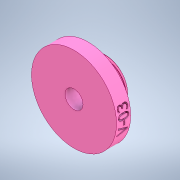
# Autodesk Inventor part: brakeHandle
Saved by Autodesk Inventor 2021.1 (Build 251245010, 245A)
## iProperties
Created: 2020-08-18
Part Number: brakeHandle
Material: Polycarbonate, Smoke
Document SubType Name: Modeling
Designer: robst
Density: 1.2 g/cm^3
Appearance: Pink
innerDiameter: 0.635 in
heightOfBrake: 0.250 in
majorDiameter: 1.623 in
pitchDiameter: 1.569 in
minorDiameter: 1.524 in
pitch: 0.083 in
crestFlat: 0.017 in
rootRadius: 0.009 in
threadsPerInch: 12.000 ul
threadDepth: 0.060 in
Author: robst
Autodesk Inventor part; units mm, degrees
ref_plane "XZ Plane" through (0, 0, 0) normal (0, 1, 0) x (-1, 0, 0)
ref_plane "XY Plane" through (0, 0, 0) normal (0, 0, 1) x (1, 0, 0)
sketch "Sketch1" plane through (0, 0, 0) normal (0, 0, 1) x (1, 0, 0)
  circle A0 centre (0, 0) radius 8.0645
  circle A1 centre (0, 0) radius 20.5061
  dimension "d0" = 16.129
  dimension "d1" = 41.0121
  constraints: 2 centre point, 2 coincident
  measures "d0" diameter of A0
  measures "d1" diameter of A1
extrude "Extrusion1" add sketch "Sketch1" against normal blind 15.24
sketch "Sketch2" plane through (0, 0, 0) normal (0, 0, 1) x (1, 0, 0)
  circle A0 centre (0, 0) radius 8.0645
  circle A1 centre (0, 0) radius 38.1
  dimension "d4" = 76.2
  dimension "d56" = 16.129
  constraints: 2 centre point, 2 coincident
  measures "d4" diameter of A1
  measures "d56" diameter of A0
extrude "Extrusion2" add sketch "Sketch2" along normal blind 12.7
sketch "Sketch9" plane through (0, 0, 0) normal (1, 0, 0) x (0, 1, 0)
  line L0 (20.5061, 0) -> (20.5061, -15.24) projected
  line L1 (-20.5061, -15.24) -> (20.5061, -15.24) projected
  line L2 (20.5061, -17.3567) -> (19.3002, -18.0529)
  line L3 (19.3002, -18.44) -> (20.5061, -19.1362)
  arc A0 (19.3002, -18.0529) -> (19.3002, -18.44) centre (19.412, -18.2464) ccw
  line L4 (20.5061, -17.3567) -> (20.5061, -19.1362)
  line L5 (0, -15.24) -> (0, -43.7839) construction
  point P0 (0, 0)
  dimension "d38" = 60
  dimension "d39" = 0.2235
  dimension "d41" = 2.1167
  dimension "d42" = 20.506
  dimension "d52" = 19.1884
  constraints: 8 end point, 2 point on circle, 2 tangent, 2 vertical, 1 centre point, 1 equal length, 1 midpoint
  measures "d38" angle of L3 L2
  measures "d39" radius of A0
  measures "d41" distance from line of L2.start L1
  measures "d42" distance from line of L4 point (0, 0)
  measures "d52" distance edge to line of A0 L5
coil "Coil2" sketch "Sketch9" operation cut axis through (0, 0, -10) along (0, 0, 1) pitch 2.1167 turns 9.2 hand right
ref_plane "Work Plane1" through (38.1, 0, 0) normal (1, 0, 0) x (0, 1, 0)
sketch "Sketch10" plane through (38.1, 0, 0) normal (1, 0, 0) x (0, 1, 0)
  line L0 (38.1, 0) -> (38.1, 12.7) construction
  line L1 (38.1, 6.35) -> (-38.1, 6.35) construction
  line L2 (-38.1, 0) -> (-38.1, 12.7) construction
  line L3 (-5.1906, 10.795) -> (-8.2524, 1.905)
  line L4 (-8.2524, 1.905) -> (-9.5276, 1.905)
  line L5 (-9.5276, 1.905) -> (-12.5894, 10.795)
  line L6 (-12.5894, 10.795) -> (-11.3214, 10.795)
  line L7 (-11.3214, 10.795) -> (-8.8576, 3.4107)
  line L8 (-8.8576, 3.4107) -> (-6.3937, 10.795)
  line L9 (-6.3937, 10.795) -> (-5.1906, 10.795)
  line L10 (-1.2355, 5.255) -> (-4.5999, 5.255)
  line L11 (-4.5999, 5.255) -> (-4.5999, 6.3356)
  line L12 (-4.5999, 6.3356) -> (-1.2355, 6.3356)
  line L13 (-1.2355, 6.3356) -> (-1.2355, 5.255)
  spline S0 degree 2 poles (5.4788, 6.35) (5.4788, 3.9582) (4.0884, 1.7177) (2.6403, 1.7177) knots 0 0 0 1 2 2 2
  spline S1 degree 2 poles (2.6403, 1.7177) (1.1707, 1.7177) (-0.2053, 4.0014) (-0.2053, 6.3428) knots 0 0 0 1 2 2 2
  spline S2 degree 2 poles (-0.2053, 6.3428) (-0.2053, 8.749) (1.1851, 10.9751) (2.6403, 10.9751) knots 0 0 0 1 2 2 2
  spline S3 degree 2 poles (2.6403, 10.9751) (4.1028, 10.9751) (5.4788, 8.6698) (5.4788, 6.35) knots 0 0 0 1 2 2 2
  spline S4 degree 2 poles (3.9515, 3.6412) (4.1244, 4.0807) (4.2685, 5.4351) (4.2685, 6.35) knots 0 0 0 1 2 2 2
  spline S5 degree 2 poles (4.2685, 6.35) (4.2685, 7.2649) (4.1244, 8.6121) (3.9443, 9.066) knots 0 0 0 1 2 2 2
  spline S6 degree 2 poles (3.9443, 9.066) (3.7642, 9.5199) (3.1374, 9.9881) (2.6403, 9.9881) knots 0 0 0 1 2 2 2
  spline S7 degree 2 poles (2.6403, 9.9881) (2.1433, 9.9881) (1.5021, 9.5199) (1.3148, 9.0516) knots 0 0 0 1 2 2 2
  spline S8 degree 2 poles (1.3148, 9.0516) (1.1347, 8.5977) (1.005, 7.2145) (1.005, 6.3428) knots 0 0 0 1 2 2 2
  spline S9 degree 2 poles (1.005, 6.3428) (1.005, 5.4062) (1.1203, 4.1527) (1.3076, 3.6628) knots 0 0 0 1 2 2 2
  spline S10 degree 2 poles (1.3076, 3.6628) (1.4805, 3.2018) (2.1216, 2.7047) (2.6403, 2.7047) knots 0 0 0 1 2 2 2
  spline S11 degree 2 poles (2.6403, 2.7047) (3.1302, 2.7047) (3.7714, 3.1729) (3.9515, 3.6412) knots 0 0 0 1 2 2 2
  spline S12 degree 2 poles (9.0161, 9.9521) (8.6919, 9.9521) (8.0507, 9.7936) (7.7409, 9.6711) knots 0 0 0 1 2 2 2
  spline S13 degree 2 poles (7.7409, 9.6711) (7.4528, 9.5487) (7.0277, 9.2893) (6.862, 9.1741) knots 0 0 0 1 2 2 2
  line L14 (6.862, 9.1741) -> (6.79, 9.1741)
  line L15 (6.79, 9.1741) -> (6.79, 10.4348)
  spline S14 degree 2 poles (6.79, 10.4348) (7.179, 10.6437) (8.5118, 10.9823) (9.1097, 10.9823) knots 0 0 0 1 2 2 2
  spline S15 degree 2 poles (9.1097, 10.9823) (9.7149, 10.9823) (10.6154, 10.7374) (10.9828, 10.478) knots 0 0 0 1 2 2 2
  spline S16 degree 2 poles (10.9828, 10.478) (11.3719, 10.1971) (11.7753, 9.383) (11.7753, 8.8355) knots 0 0 0 1 2 2 2
  spline S17 degree 2 poles (11.7753, 8.8355) (11.7753, 8.1006) (10.8099, 6.9912) (10.1327, 6.8471) knots 0 0 0 1 2 2 2
  line L16 (10.1327, 6.8471) -> (10.1327, 6.7606)
  spline S18 degree 2 poles (10.1327, 6.7606) (10.4137, 6.703) (11.0549, 6.4437) (11.3286, 6.1843) knots 0 0 0 1 2 2 2
  spline S19 degree 2 poles (11.3286, 6.1843) (11.6024, 5.9322) (11.9482, 5.1253) (11.9482, 4.5417) knots 0 0 0 1 2 2 2
  spline S20 degree 2 poles (11.9482, 4.5417) (11.9482, 3.9438) (11.5375, 2.928) (11.1629, 2.539) knots 0 0 0 1 2 2 2
  spline S21 degree 2 poles (11.1629, 2.539) (10.7739, 2.1355) (9.6717, 1.7177) (8.9728, 1.7177) knots 0 0 0 1 2 2 2
  spline S22 degree 2 poles (8.9728, 1.7177) (8.3029, 1.7177) (6.9917, 2.0419) (6.545, 2.2652) knots 0 0 0 1 2 2 2
  line L17 (6.545, 2.2652) -> (6.545, 3.5259)
  line L18 (6.545, 3.5259) -> (6.6315, 3.5259)
  spline S23 degree 2 poles (6.6315, 3.5259) (7.0061, 3.2522) (8.274, 2.7479) (8.9008, 2.7479) knots 0 0 0 1 2 2 2
  spline S24 degree 2 poles (8.9008, 2.7479) (9.2682, 2.7479) (10.0031, 2.9784) (10.248, 3.245) knots 0 0 0 1 2 2 2
  spline S25 degree 2 poles (10.248, 3.245) (10.4857, 3.5115) (10.7379, 4.1455) (10.7379, 4.6282) knots 0 0 0 1 2 2 2
  spline S26 degree 2 poles (10.7379, 4.6282) (10.7379, 5.1109) (10.4569, 5.7376) (10.2048, 5.9177) knots 0 0 0 1 2 2 2
  spline S27 degree 2 poles (10.2048, 5.9177) (9.9526, 6.0979) (9.2682, 6.2347) (8.8648, 6.2347) knots 0 0 0 1 2 2 2
  line L19 (8.8648, 6.2347) -> (8.3605, 6.2347)
  line L20 (8.3605, 6.2347) -> (8.3605, 7.2217)
  line L21 (8.3605, 7.2217) -> (8.7567, 7.2217)
  spline S28 degree 2 poles (8.7567, 7.2217) (9.5564, 7.2217) (10.565, 7.9854) (10.565, 8.713) knots 0 0 0 1 2 2 2
  spline S29 degree 2 poles (10.565, 8.713) (10.565, 9.0516) (10.3056, 9.5343) (10.0967, 9.6783) knots 0 0 0 1 2 2 2
  spline S30 degree 2 poles (10.0967, 9.6783) (9.8734, 9.8296) (9.3259, 9.9521) (9.0161, 9.9521) knots 0 0 0 1 2 2 2
  point P0 (0, 0)
  constraints: 2 end point, 2 midpoint, 1 horizontal
emboss "Emboss1" sketch "Sketch10" operation cut depth 2.54 direction (-1, 0, 0) wrap yes faces at (37.6745, -5.6785, 8.4667)
equation "\"d0\" = innerDiameter"
equation "\"d1\" = a1MajorDiameterAvg"
equation "\"d2\" = threadPostLength"
equation "\"d4\" = handleDiameter"
equation "\"d56\" = innerDiameter"
equation "\"d5\" = handleLength"
equation "\"d39\" = rootRadius"
equation "\"d41\" = pitch"
equation "\"d42\" = 0.5 * a1MajorDiameterAvg"
equation "\"d52\" = 0.5 * a1MinorDiameterAvg"
equation "\"d43\" = pitch"
equation "\"d44\" = threadLength"
equation "\"handleDiameter\" = 76.2"
equation "\"brakeHandle\" = 30deg"
equation "\"innerDiameter\" = 16.129"
equation "\"heightOfBrake\" = 6.35"
equation "\"majorDiameter\" = 41.22928"
equation "\"pitchDiameter\" = 39.85514"
equation "\"minorDiameter\" = 38.7096"
equation "\"crestFlat\" = 0.4318"
equation "\"rootRadius\" = 0.22352"
equation "\"threadsPerInch\" = 12"
equation "\"threadDepth\" = 1.52146"
equation "\"d53\" = 0.5 * handleDiameter"
equation "\"totalLength\" = 27.94"
equation "\"handleLength\" = 12.7"
equation "\"threadPostLength\" = totalLength - handleLength"
equation "\"threadLength\" = threadPostLength + 2 * pitch"
equation "\"brakeStopLength\" = 12.7"
equation "\"a1MajorDiameterMax\" = 41.22928"
equation "\"a1MajorDiameterMin\" = 40.79494"
equation "\"a1MajorDiameterAvg\" = 0.5 * a1MajorDiameterMin + 0.5 * a1MajorDiameterMax"
equation "\"a1MinorDiameterMax\" = 38.7096"
equation "\"a1MinorDiameterMin\" = 38.04412"
equation "\"a1MinorDiameterAvg\" = 0.5 * a1MinorDiameterMin + 0.5 * a1MinorDiameterMax"
equation "\"a1RootRadiusMax\" = 0.26162"
equation "\"a1RootRadiusMin\" = 0.1524"
equation "\"a1RootRadiusAvg\" = 0.5 * a1RootRadiusMin + 0.5 * a1RootRadiusMax"
equation "\"pitch\" = 2.116667"
body "Solid1"
